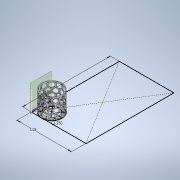
# Autodesk Inventor part: pokerChipsHolder_20r50h
Saved by Autodesk Inventor 2020 (Build 240168000, 168)
## iProperties
Created: 2021-04-19
Part Number: pokerChipsHolder_20r50h
Material: Generic
Document SubType Name: Modeling
Designer: Vlasciar
Density: 1 g/cm^3
Appearance: Default
Author: Vlasciar
Autodesk Inventor part; units mm, degrees
ref_plane "YZ Plane" through (0, 0, 0) normal (1, 0, 0) x (0, 1, 0)
ref_plane "XZ Plane" through (0, 0, 0) normal (0, 1, 0) x (-1, 0, 0)
ref_plane "XY Plane" through (0, 0, 0) normal (0, 0, 1) x (1, 0, 0)
sketch "Sketch1" plane through (0, 0, 0) normal (0, 1, 0) x (-1, 0, 0)
  line L0 (-57.5, -92.5) -> (57.5, -92.5)
  line L1 (57.5, -92.5) -> (57.5, 92.5)
  line L2 (57.5, 92.5) -> (-57.5, 92.5)
  line L3 (-57.5, 92.5) -> (-57.5, -92.5)
  line L4 (-57.5, -92.5) -> (57.5, 92.5) construction
  line L5 (57.5, -92.5) -> (-57.5, 92.5) construction
  circle A0 centre (36, 71) radius 21.5
  circle A1 centre (36, 71) radius 20.25
  circle A2 centre (36, 71) radius 15
  point P0 (0, 0)
  point P1 (57.5, 71)
  dimension "d2" = 43
  dimension "d0" = 115
  dimension "d1" = 185
  dimension "d3" = 40.5
  dimension "d6" = 30
  dimension "d41" = 1.25
  constraints: 12 end point, 2 centre point, 2 coincident, 2 horizontal, 2 midpoint, 2 parallel, 1 horizontal alignment, 1 perpendicular, 1 point on line, 1 vertical, 2 other
  measures "d0" distance of L1.end L2.end
  measures "d1" distance of L0.end L1.end
  measures "d3" diameter of A1
  measures "d6" diameter of A2
extrude "Extrusion1" add sketch "Sketch1" along normal blind 1 contours A1
extrude "Extrusion2" add sketch "Sketch1" along normal blind 42 contours A0
ref_plane "Work Plane1" through (-57.5, 0, -92.5) normal (-1, 0, 0) x (0, -1, 0)
sketch "Sketch2" plane through (-57.5, 0, -92.5) normal (-1, 0, 0) x (0, -1, 0)
  line L0 (0, 142) -> (-42, 142) projected
  line L1 (0, 185) -> (-42, 185) projected
  line L2 (0, 165) -> (-2.75, 160.2369)
  line L3 (-2.75, 160.2369) -> (-8.25, 160.2369)
  line L4 (-8.25, 160.2369) -> (-11, 165)
  line L5 (-11, 165) -> (-8.25, 169.7631)
  line L6 (-8.25, 169.7631) -> (-2.75, 169.7631)
  line L7 (-2.75, 169.7631) -> (0, 165)
  line L8 (0, 148.5) -> (0, 178.5) projected
  line L9 (0, 163.1291) -> (0, 167)
  line L10 (-2.2685, 142) -> (-2.2685, 161.0708)
  line L11 (-2.2685, 168.9292) -> (-2.2685, 185)
  point P0 (0, 92.5)
  point P1 (-2.2685, 165)
  point P2 (-5.5, 165)
  point P3 (0, 163.5)
  point P4 (0, 165.0646)
  dimension "d11" = 5.5
  constraints: 18 end point, 6 point on line, 2 midpoint, 2 vertical, 1 vertical alignment, 13 other
  measures "d11" distance of L2.start point (-5.5, 165)
extrude "Extrusion3" cut sketch "Sketch2" against normal blind 6
pattern_circular "Circular Pattern1" count 11 over 360 about axis through (-36, 0, 71) along (0, 1, 0) of "Extrusion3"
sketch "Sketch3" plane through (-57.5, 0, -92.5) normal (-1, 0, 0) x (0, -1, 0)
  line L0 (-10, 159.5) -> (-12.75, 154.7369)
  line L1 (-12.75, 154.7369) -> (-18.25, 154.7369)
  line L2 (-18.25, 154.7369) -> (-21, 159.5)
  line L3 (-21, 159.5) -> (-18.25, 164.2631)
  line L4 (-18.25, 164.2631) -> (-12.75, 164.2631)
  line L5 (-12.75, 164.2631) -> (-10, 159.5)
  line L6 (-11, 165) -> (-8.25, 160.2369) projected
  line L7 (0, 183.6326) -> (0, 144.6137) projected
  point P0 (0, 92.5)
  point P1 (-15.5, 159.5)
  dimension "d34" = 5.5
  dimension "d35" = 10
  dimension "d36" = 5.5
  constraints: 12 end point, 1 vertical alignment, 13 other
  measures "d34" distance of L2.end point (-15.5, 159.5)
  measures "d35" distance from line of L7 L0.start
  measures "d36" vertical distance of L6.start L0.start
extrude "Extrusion4" cut sketch "Sketch3" along normal mid plane 8
pattern_circular "Circular Pattern2" count 11 over 360 about axis through (-36, 0, 71) along (0, 1, 0) of "Extrusion4"
pattern_linear "Rectangular Pattern1" count 3 spacing 19.5 along (0, 1, 0) of "Extrusion3", "Circular Pattern1"
sketch "Sketch4" plane through (-36, 42, 71) normal (0, 1, 0) x (1, 0, 0)
  circle A0 centre (0, 0) radius 21.5 projected
  circle A1 centre (0, 0) radius 20.25 projected
  point P0 (36, 71)
pattern_linear "Rectangular Pattern2" count 3 spacing 19.5 along (0, 1, 0) of "Extrusion4", "Circular Pattern2"
extrude "Extrusion5" add sketch "Sketch4" against normal blind 2
extrude "Extrusion6" add sketch "Sketch1" along normal blind 1 contours A0 | A1
extrude "Extrusion7" add sketch "Sketch1" against normal blind 1.5 contours A0 | A1 | A2
extrude "Extrusion8" cut sketch "Sketch1" against normal blind 8 contours A2
body "Solid1"
